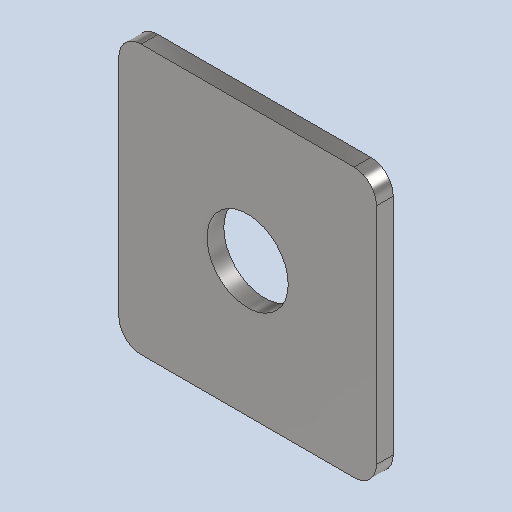
# Autodesk Inventor part: NDM 4.0.2  base plate
Saved by Autodesk Inventor 2025 (Build 290162010, 162A)
## iProperties
Created: 2023-07-04
Part Number: NDM 4.0.2  base plate
Material: Stainless Steel
Document SubType Name: Sheet Metal
Designer: user
Density: 8 g/cm^3
Sheet Metal Rule: Default
Appearance: Semi-Polished
Stock Number: NDM 4.0.2 основание домкрата
Flat Pattern Width: 4.6 cm
Flat Pattern Length: 4.8 cm
Flat Pattern Area: 22.08 cm^2
Sheet Metal Width: 46,000 mm
Sheet Metal Length: 48,000 mm
Sheet Metal Area: 2208,000 mm^2
Description: лист 3mm
Mass: 48.6993 g
Surface Area: 47.3833 cm^2
Volume: 6.08741 cm^3
Author: user
Revision Number: 1
Autodesk Inventor part; units mm, degrees
ref_plane "YZ Plane" through (0, 0, 0) normal (1, 0, 0) x (0, 1, 0)
ref_plane "XZ Plane" through (0, 0, 0) normal (0, 1, 0) x (-1, 0, 0)
ref_plane "XY Plane" through (0, 0, 0) normal (0, 0, 1) x (1, 0, 0)
sketch "Sketch1" plane through (0, 0, 0) normal (0, 0, 1) x (1, 0, 0)
  line L0 (-23, -24) -> (23, -24)
  line L1 (23, -24) -> (23, 24)
  line L2 (23, 24) -> (-23, 24)
  line L3 (-23, 24) -> (-23, -24)
  line L4 (-23, -24) -> (23, 24) construction
  line L5 (23, -24) -> (-23, 24) construction
  point P0 (0, 0)
  dimension "d0" = 46
  dimension "d1" = 48
  constraints: 12 end point, 2 midpoint, 2 parallel, 1 horizontal, 1 perpendicular
  measures "d0" distance of L2.end L1.end
  measures "d1" distance of L1.end L0.end
extrude "Plate1" add sketch "Sketch1" along normal blind 3
fillet "Corner Round1" radius 4 4 edges at (23, -24, 1.5) (23, 24, 1.5) (-23, -24, 1.5) (-23, 24, 1.5)
sketch "Sketch2" plane through (0, 0, 3) normal (0, 0, 1) x (1, 0, 0)
  circle A0 centre (0, 0) radius 7.25
  dimension "d4" = 14.5
  constraints: 1 centre point, 1 coincident
  measures "d4" diameter of A0
extrude "Extrusion1" cut sketch "Sketch2" against normal through all
equation "\"d2\" = Thickness"
equation "\"BendRadius\" = Thickness"
equation "\"BendReliefWidth\" = Thickness"
equation "\"BendReliefDepth\" = 0.5 * Thickness"
equation "\"CornerReliefSize\" = 4 * Thickness"
equation "\"MinimumRemnant\" = 2 * Thickness"
equation "\"TransitionRadius\" = BendRadius"
equation "\"JacobiRadiusSize\" = BendRadius"
equation "\"GapSize\" = Thickness"
equation "\"Thickness\" = 3"
body "Solid1"
